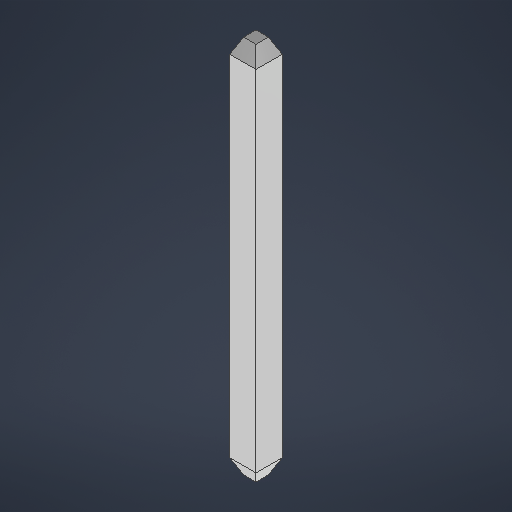
# Autodesk Inventor part: Pin_Header
Saved by Autodesk Inventor 2026 (Build 300175000, 175)
## iProperties
Created: 2025-04-18
Part Number: Pin_Header
Material: Nickel-Copper Alloy 400
Document SubType Name: Modeling
Designer: ct_vi
Density: 8.83 g/cm^3
Appearance: Chrome - Polished
Author: ct_vi
Autodesk Inventor part; units mm, degrees
ref_plane "YZ Plane" through (0, 0, 0) normal (1, 0, 0) x (0, 1, 0)
ref_plane "XZ Plane" through (0, 0, 0) normal (0, 1, 0) x (-1, 0, 0)
ref_plane "XY Plane" through (0, 0, 0) normal (0, 0, 1) x (1, 0, 0)
sketch "Sketch1" plane through (0, 0, 0) normal (1, 0, 0) x (0, 1, 0)
  line L0 (4.475, 0.31) -> (-4.475, 0.31)
  line L1 (-4.475, 0.31) -> (-4.475, -0.31)
  line L2 (-4.475, -0.31) -> (4.475, -0.31)
  line L3 (4.475, -0.31) -> (4.475, 0.31)
  line L4 (4.475, 0.31) -> (-4.475, -0.31) construction
  line L5 (-4.475, 0.31) -> (4.475, -0.31) construction
  point P0 (0, 0)
  dimension "d0" = 8.95
  dimension "d1" = 0.62
  constraints: 12 end point, 2 midpoint, 2 parallel, 1 horizontal, 1 perpendicular
  measures "d0" distance of L2.end L1.end
  measures "d1" distance of L1.end L0.end
extrude "Extrusion1" add sketch "Sketch1" along normal blind 0.62
chamfer "Chamfer1" distance 0.35 angle 25 1 edges at (0.31, 4.475, 0.31) measured on face at (0.4133, 1.4917, 0.31)
chamfer "Chamfer2" distance 0.35 angle 25 1 edges at (0.62, 4.475, -0.0816) measured on face at (0.62, 1.375, -0.1033)
chamfer "Chamfer3" distance 0.35 angle 25 1 edges at (0.2284, 4.475, -0.31) measured on face at (0.2067, 1.375, -0.31)
chamfer "Chamfer4" distance 0.35 angle 25 1 edges at (0, 4.475, 0) measured on face at (0, 1.2583, -0.1033)
chamfer "Chamfer5" distance 0.35 angle 25 1 edges at (0.31, -4.475, -0.31) measured on face at (0.2067, -1.6083, -0.31)
chamfer "Chamfer6" distance 0.35 angle 25 1 edges at (0.62, -4.475, 0.0816) measured on face at (0.62, -1.4917, 0.1033)
chamfer "Chamfer7" distance 0.35 angle 25 1 edges at (0.2284, -4.475, 0.31) measured on face at (0.2067, -1.4917, 0.31)
chamfer "Chamfer8" distance 0.35 angle 25 1 edges at (0, -4.475, 0) measured on face at (0, 1.375, -0.1033)
body "Solid1"
